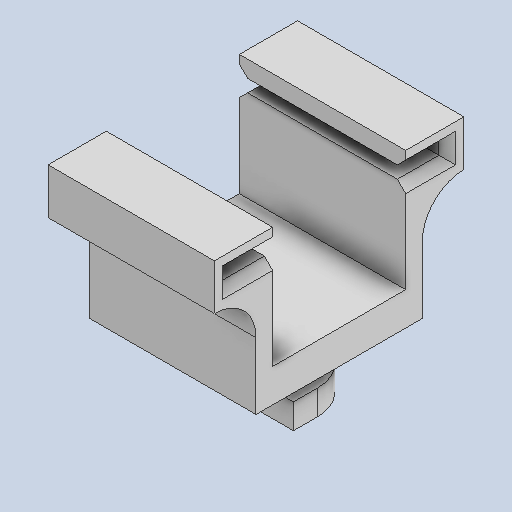
# Autodesk Inventor part: Drziak_4
Saved by Autodesk Inventor 2025 (Build 290162000, 162)
## iProperties
Created: 2025-06-09
Part Number: Drziak_4
Material: Generic
Document SubType Name: Modeling
Designer: Pravoslav
Density: 1 g/cm^3
Appearance: Default
Author: Pravoslav
Autodesk Inventor part; units mm, degrees
ref_plane "YZ Plane" through (0, 0, 0) normal (1, 0, 0) x (0, 1, 0)
ref_plane "XZ Plane" through (0, 0, 0) normal (0, 1, 0) x (-1, 0, 0)
ref_plane "XY Plane" through (0, 0, 0) normal (0, 0, 1) x (1, 0, 0)
sketch "Sketch1" plane through (0, 0, 0) normal (1, 0, 0) x (0, 1, 0)
  line L0 (0, 8) -> (0, -8)
  line L1 (0, -8) -> (11, -8)
  line L2 (0, 8) -> (11, 8)
  line L3 (11, 8) -> (11, 13)
  line L4 (11, 13) -> (12.5, 13)
  line L5 (12.5, 13) -> (12.5, 8)
  line L6 (12.5, 8) -> (14.5, 8)
  line L7 (14.5, 8) -> (14.5, 15)
  line L8 (14.5, 15) -> (9, 15)
  line L9 (9, 15) -> (9, 10)
  line L10 (9, 10) -> (-3, 10)
  line L11 (-3, 10) -> (-4, 10)
  line L12 (-4, 10) -> (-4, 2.5)
  line L13 (0, 0) -> (3.5, 0)
  line L14 (0, -8) -> (11, -8)
  line L15 (11, -8) -> (11, -13)
  line L16 (11, -13) -> (12.5, -13)
  line L17 (12.5, -13) -> (12.5, -8)
  line L18 (14.5, -8) -> (14.5, -15)
  line L19 (14.5, -15) -> (9, -15)
  line L20 (9, -15) -> (9, -10)
  line L21 (9, -10) -> (-3, -10)
  line L22 (-3, -10) -> (-4, -10)
  line L23 (-4, -10) -> (-4, 2.5)
  line L24 (14.5, -8) -> (12.5, -8)
  point P0 (11.75, -15)
  point P1 (11.75, -13)
  dimension "d0" = 16
  dimension "d1" = 0
  dimension "d2" = 11
  dimension "d3" = 11
  dimension "d4" = 5
  dimension "d5" = 1.5
  dimension "d6" = 2
  dimension "d7" = 7
  dimension "d8" = 5.5
  dimension "d9" = 5
  dimension "d10" = 1
  dimension "d13" = 2
  dimension "d14" = 4
  constraints: 50 end point, 9 symmetric about line, 8 perpendicular, 4 horizontal, 3 midpoint, 2 point on line, 2 vertical
  measures "d0" distance of L0.start L0.end
  measures "d1" distance of point (0, 0) L13.start
  measures "d2" distance of L0.end L1.end
  measures "d3" distance of L0.start L2.end
  measures "d4" distance of L2.end L3.end
  measures "d5" distance of L3.end L4.end
  measures "d6" distance of L5.end L6.end
  measures "d7" distance of L6.end L7.end
  measures "d8" distance of L7.end L8.end
  measures "d9" distance of L8.end L9.end
  measures "d10" distance of L10.end L11.end
  measures "d13" distance of point (11.75, -15) point (11.75, -13)
  measures "d14" distance between parallel lines of L23 L0
extrude "Extrusion1" add sketch "Sketch1" along normal blind 20
fillet "Fillet1" radius 5 2 edges at (10, 9, -10) (10, 9, 10)
chamfer "Chamfer1" distance 1 angle 45 12 edges at (20, 11, -10.5) (20, 11.75, -13) (20, 12.5, -10.5) (20, 11, 10.5) (20, 11.75, 13) (20, 12.5, 10.5) (0, 11, -10.5) (0, 11.75, -13) (0, 12.5, -10.5) (0, 11, 10.5) (0, 11.75, 13) (0, 12.5, 10.5)
sketch "Sketch3" plane through (0, -4, -10) normal (0, -1, 0) x (1, 0, 0)
  line L0 (13.95, 6.05) -> (6.05, 6.05)
  line L1 (6.05, 6.05) -> (6.05, 13.95)
  line L2 (6.05, 13.95) -> (13.95, 13.95)
  line L3 (13.95, 13.95) -> (13.95, 6.05)
  line L4 (20, 20) -> (20, 0) projected
  line L5 (0, -5) -> (20, -5) projected
  point P0 (0, 10)
  point P1 (20, 10)
  dimension "d28" = 7.9
  dimension "d29" = 7.9
  dimension "d30" = 6.05
  dimension "d31" = 11.05
  constraints: 8 end point, 2 parallel, 1 horizontal, 1 midpoint, 1 perpendicular
  measures "d28" distance of L1.end L2.end
  measures "d29" distance of L0.end L1.end
  measures "d30" distance from line of point (20, 10) L3
  measures "d31" distance between parallel lines of L5 L0
extrude "Extrusion3" add sketch "Sketch3" along normal blind 2.49
sketch "Sketch4" plane through (0, -6.49, -10) normal (0, -1, 0) x (1, 0, 0)
  line L0 (18.45, 6.05) -> (1.55, 6.05)
  line L1 (1.55, 6.05) -> (1.55, 13.95)
  line L2 (1.55, 13.95) -> (18.45, 13.95)
  line L3 (18.45, 13.95) -> (18.45, 6.05)
  line L4 (6.05, 6.05) -> (13.95, 6.05) projected
  line L5 (13.95, 13.95) -> (6.05, 13.95) projected
  line L6 (20, 20) -> (20, 0) projected
  point P0 (0, 10)
  point P1 (18.45, 10)
  dimension "d34" = 0
  dimension "d35" = 0
  dimension "d36" = 16.9
  dimension "d37" = 1.55
  constraints: 8 end point, 2 parallel, 1 horizontal, 1 midpoint, 1 perpendicular
  measures "d34" distance between parallel lines of L4 L0
  measures "d35" distance between parallel lines of L5 L2
  measures "d36" distance from line of L1 point (18.45, 10)
  measures "d37" distance between parallel lines of L6 L3
extrude "Extrusion4" add sketch "Sketch4" along normal blind 3
fillet "Fillet2" radius 5 4 edges at (18.45, -7.99, -3.95) (13.95, -5.245, -3.95) (6.05, -5.245, 3.95) (1.55, -7.99, 3.95)
sketch "Sketch2" plane through (0, 0, 8) normal (0, 1, 0) x (1, 0, 0)
  circle A0 centre (10, 7.5) radius 3
  line L0 (20, 16) -> (20, 0) projected
  line L1 (0, -7) -> (20, -7) projected
  line L2 (0, 0) -> (20, 0) projected
  point P0 (0, 8)
  dimension "d19" = 6
  dimension "d20" = 10
  dimension "d27" = 7.5
  constraints: 1 centre point
  measures "d19" diameter of A0
  measures "d20" distance from line of L0 A0.centre
  measures "d27" distance from line of L2 A0.centre
body "Solid1"
